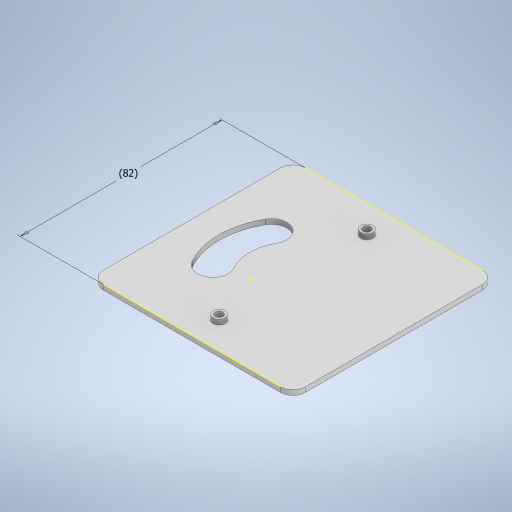
# Autodesk Inventor part: controler_01
Saved by Autodesk Inventor 2023 (Build 270158000, 158)
## iProperties
Created: 2023-10-09
Part Number: controler_01
Material: Generic
Document SubType Name: Modeling
Designer: Michal
Density: 1 g/cm^3
Appearance: Default
Author: Michal
Autodesk Inventor part; units mm, degrees
ref_plane "YZ Plane" through (0, 0, 0) normal (1, 0, 0) x (0, 1, 0)
ref_plane "XZ Plane" through (0, 0, 0) normal (0, 1, 0) x (-1, 0, 0)
ref_plane "XY Plane" through (0, 0, 0) normal (0, 0, 1) x (1, 0, 0)
sketch "Sketch1" plane through (0, 0, 0) normal (0, 1, 0) x (-1, 0, 0)
  line L0 (32.8496, 31.7326) -> (-49.1504, 31.7326)
  line L1 (-49.1504, 31.7326) -> (-49.1504, -50.2674)
  line L2 (-49.1504, -50.2674) -> (32.8496, -50.2674)
  line L3 (32.8496, -50.2674) -> (32.8496, 31.7326)
  circle A0 centre (-8.1504, -9.2674) radius 30
  circle A1 centre (-8.1504, -39.2674) radius 2.5
  circle A2 centre (-8.1504, 20.7326) radius 2.5
  circle A3 centre (-8.1504, -39.2674) radius 1.6
  circle A4 centre (-8.1504, 20.7326) radius 1.6
  arc A5 (12.448, -21.16) -> (12.4481, 2.625) centre (-8.1504, -9.2674) ccw construction
  arc A6 (17.8304, -24.2675) -> (17.8305, 5.7325) centre (-8.1504, -9.2674) ccw
  arc A7 (7.0656, -18.0524) -> (7.0657, -0.4825) centre (-8.1504, -9.2674) ccw
  arc A8 (7.0656, -18.0524) -> (17.8304, -24.2675) centre (12.448, -21.16) ccw
  arc A9 (17.8305, 5.7325) -> (7.0657, -0.4825) centre (12.4481, 2.625) ccw
  line L4 (-8.1504, -9.2674) -> (12.448, -21.16) construction
  line L5 (-8.1504, -9.2674) -> (12.4481, 2.625) construction
  point P0 (0, 0)
  point P1 (17.8304, -24.2675)
  point P2 (17.8305, 5.7325)
  dimension "d0" = 82
  dimension "d1" = 82
  dimension "d2" = 60
  dimension "d3" = 5
  dimension "d4" = 5
  dimension "d5" = 3.2
  dimension "d6" = 3.2
  dimension "d7" = 60
  constraints: 13 point on circle, 12 end point, 10 centre point, 5 coincident, 4 tangent, 2 parallel, 1 concentric, 1 horizontal, 1 perpendicular
  measures "d0" distance of L2.end L0.start
  measures "d1" distance of L1.end L2.end
  measures "d2" diameter of A0
  measures "d3" diameter of A1
  measures "d4" diameter of A2
  measures "d5" diameter of A3
  measures "d6" diameter of A4
  measures "d7" angle of L4 L5
extrude "Extrusion1" add sketch "Sketch1" along normal blind 2 contours L3 L2 L1 L0 | A9 A7 A8 A0 A1 A2
extrude "Extrusion2" add sketch "Sketch1" along normal blind 4 contours A2 A0 A4 | A0 A4 A2 | A1 A0 A3 | A0 A3 A1
sketch "Sketch2" plane through (0, 2, 0) normal (0, 1, 0) x (1, 0, 0)
  line L0 (49.1504, -31.7326) -> (49.1504, 50.2674) projected
  line L1 (49.1504, 50.2674) -> (-32.8496, 50.2674) projected
  line L2 (-32.8496, 50.2674) -> (-32.8496, -31.7326) projected
  line L3 (-32.8496, -31.7326) -> (49.1504, -31.7326) projected
  circle A0 centre (8.1504, -20.7326) radius 2.5 projected
  circle A1 centre (8.1504, 39.2674) radius 2.5 projected
  arc A2 (-7.0656, 18.0524) -> (-17.8304, 24.2675) centre (-12.448, 21.16) ccw projected
  arc A3 (-7.0656, 18.0524) -> (-7.0657, 0.4825) centre (8.1504, 9.2674) ccw projected
  arc A4 (-17.8305, -5.7325) -> (-7.0657, 0.4825) centre (-12.4481, -2.625) ccw projected
  arc A5 (-17.8304, 24.2675) -> (-17.8305, -5.7325) centre (8.1504, 9.2674) ccw projected
  circle A6 centre (-27.8496, 45.2674) radius 5
  circle A7 centre (-27.8496, -26.7326) radius 5
  circle A8 centre (44.1504, 45.2674) radius 5
  circle A9 centre (44.1504, -26.7326) radius 5
  point P0 (0, 0)
  point P1 (-27.8496, -31.7326)
  point P2 (-32.8496, -26.7326)
  point P3 (49.1504, -26.7326)
  point P4 (44.1504, -31.7326)
  point P5 (44.1504, 50.2674)
  point P6 (49.1504, 45.2674)
  point P7 (-32.8496, 45.2674)
  point P8 (-27.8496, 50.2674)
  dimension "d12" = 10
  dimension "d13" = 0
  dimension "d14" = 0
  dimension "d15" = 10
  dimension "d16" = 0
  dimension "d17" = 10
  dimension "d18" = 0
  dimension "d19" = 10
  constraints: 4 centre point
  measures "d12" diameter of A6
  measures "d13" distance edge to line of A6 L1
  measures "d14" distance edge to line of A6 L2
  measures "d15" diameter of A7
  measures "d16" distance edge to line of A7 L3
  measures "d17" diameter of A8
  measures "d18" distance edge to line of A8 L0
  measures "d19" diameter of A9
extrude "Extrusion3" cut sketch "Sketch2" along normal mid plane 4 contours L3 A9 L0 | A8 L1 L0 | L3 L2 A7 | A6 L2 L1
sketch "Sketch3" plane through (0, 2, 0) normal (0, 1, 0) x (1, 0, 0)
  line L0 (44.1504, 50.2674) -> (-27.8496, 50.2674) projected
  line L1 (-27.8496, -31.7326) -> (44.1504, -31.7326) projected
  point P0 (0, 0)
  dimension "d22" = 82
  measures "d22" distance between parallel lines of L0 L1
body "Solid1"
